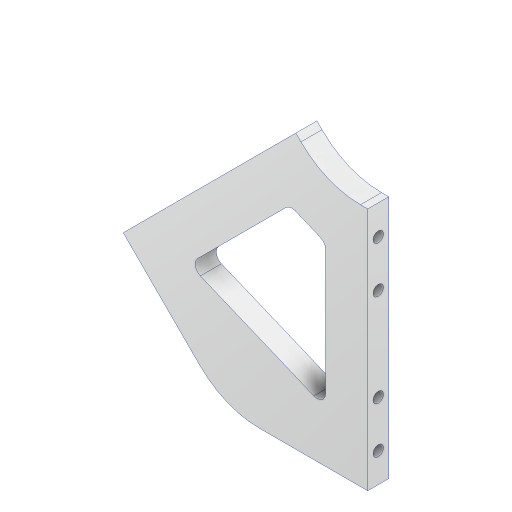
# Autodesk Inventor part: 조인트3_박스사이드_6T
Saved by Autodesk Inventor 2023.2 (Build 272271000, 271)
## iProperties
Created: 2022-01-24
Part Number: 조인트3_박스사이드_6T
Material: 알루미늄 6061
Document SubType Name: Modeling
Designer: BAEK
Density: 2.7 g/cm^3
Appearance: 알루미늄 - 평지
Mass: 29.5114 g
Surface Area: 59.5871 cm^2
Volume: 10.9301 cm^3
Author: BAEK
Autodesk Inventor part; units mm, degrees
ref_plane "YZ Plane" through (0, 0, 0) normal (1, 0, 0) x (0, 1, 0)
ref_plane "XZ Plane" through (0, 0, 0) normal (0, 1, 0) x (-1, 0, 0)
ref_plane "XY Plane" through (0, 0, 0) normal (0, 0, 1) x (1, 0, 0)
sketch "스케치1" plane through (0, 0, 0) normal (0, 0, 1) x (1, 0, 0)
  line L0 (0, 0) -> (0, 58)
  line L1 (0, 58) -> (-1.7157, 58)
  line L2 (-15.8579, 63.8579) -> (-17.0711, 65.0711)
  line L3 (-10, 58) -> (-8.2843, 58) construction
  line L4 (-17.0711, 65.0711) -> (-58.0833, 24.0589)
  line L5 (-58.0833, 24.0589) -> (-39.8823, 5.8579)
  line L6 (-25.7401, 0) -> (0, 0)
  arc A0 (-15.8579, 63.8579) -> (-1.7157, 58) centre (-1.7157, 78) ccw
  arc A1 (-39.8823, 5.8579) -> (-25.7401, 0) centre (-25.7401, 20) ccw
  point P0 (-34.0244, 0)
  dimension "d4" = 58
  dimension "d5" = 10
  dimension "d7" = 10
  dimension "d8" = 135
  dimension "d11" = 58
  dimension "d14" = 135
  dimension "d16" = 20
  dimension "d53" = 45
  constraints: 14 end point, 4 point on circle, 4 tangent, 2 centre point, 2 horizontal, 2 point on line, 1 equal length, 1 equal radius, 1 perpendicular, 1 vertical
  measures "d4" distance of L0.start L0.end
  measures "d5" distance of L0.end L3.start
  measures "d7" distance of L3.start L2.end
  measures "d8" angle of L3 L2
  measures "d11" distance of L2.end L4.end
  measures "d14" angle of L5 L6
  measures "d16" radius of A0
  measures "d53" angle of L0 L4
extrude "돌출1" add sketch "스케치1" along normal blind 5
sketch "스케치3" plane through (0, 0, 5) normal (0, 0, 1) x (1, 0, 0)
  line L0 (-19.4302, 48.5698) -> (-40.4104, 27.5896)
  line L1 (-17.0711, 65.0711) -> (-58.0833, 24.0589) projected
  line L2 (-58.0833, 24.0589) -> (-39.8823, 5.8579) projected
  line L3 (-15.8579, 63.8579) -> (-17.0711, 65.0711) projected
  line L4 (-10, 44.6636) -> (-10, 14.9932)
  line L5 (0, 58) -> (-1.7157, 58) projected
  line L6 (-25.7401, 0) -> (0, 0) projected
  line L7 (0, 0) -> (0, 58) projected
  line L8 (-39.7615, 24.3276) -> (-12.7654, 13.1455)
  line L9 (-11.2346, 46.5114) -> (-17.2506, 49.0033)
  arc A0 (-40.4104, 27.5896) -> (-39.7615, 24.3276) centre (-38.9962, 26.1754) ccw
  arc A1 (-12.7654, 13.1455) -> (-10, 14.9932) centre (-12, 14.9932) ccw
  arc A2 (-10, 44.6636) -> (-11.2346, 46.5114) centre (-12, 44.6636) ccw
  arc A3 (-17.2506, 49.0033) -> (-19.4302, 48.5698) centre (-18.016, 47.1556) ccw
  point P0 (-43.9411, 24.0589)
  point P1 (-36.8701, 16.9878)
  point P2 (-10, 10)
  point P3 (-20, 10)
  point P4 (-18.4853, 49.5147)
  point P5 (-42.5269, 25.4731)
  point P6 (-10, 46)
  point P7 (-10, 12)
  dimension "d17" = 10
  dimension "d20" = 10
  dimension "d23" = 10
  dimension "d24" = 10
  dimension "d52" = 2
  constraints: 10 point on line, 8 end point, 8 point on circle, 8 tangent, 4 centre point, 3 equal radius, 2 parallel
  measures "d17" distance between parallel lines of L1 L0
  measures "d20" distance of point (-43.941, 24.059) point (-36.87, 16.988)
  measures "d23" distance of point (-10, 10) point (-20, 10)
  measures "d24" distance between parallel lines of L7 L4
  measures "d52" radius of A0
extrude "돌출2" cut sketch "스케치3" against normal blind 6
sketch "스케치4" plane through (-58.0833, 24.0589, 0) normal (-0.7071, 0.7071, 0) x (-0.7071, -0.7071, 0)
  line L0 (-58, 0) -> (-58, 5) projected
  line L1 (-58, 2.5) -> (0, 2.5) construction
  line L2 (0, 0) -> (0, 5) projected
  circle A0 centre (-51, 2.5) radius 1.25
  circle A1 centre (-40, 2.5) radius 1.25
  circle A2 centre (-18, 2.5) radius 1.25
  circle A3 centre (-7, 2.5) radius 1.25
  point P0 (-24.0589, 0)
  dimension "d29" = 2.5
  dimension "d30" = 2.5
  dimension "d31" = 2.5
  dimension "d32" = 2.5
  dimension "d33" = 7
  dimension "d34" = 11
  dimension "d35" = 22
  dimension "d36" = 11
  constraints: 4 centre point, 4 point on line, 2 end point, 2 midpoint
  measures "d29" diameter of A0
  measures "d30" diameter of A1
  measures "d31" diameter of A2
  measures "d32" diameter of A3
  measures "d33" distance of L1.start A0.centre
  measures "d34" distance of A0.centre A1.centre
  measures "d35" distance of A1.centre A2.centre
  measures "d36" distance of A2.centre A3.centre
extrude "돌출3" cut sketch "스케치4" against normal blind 6
sketch "스케치5" plane through (0, 0, 0) normal (1, 0, 0) x (0, 0, -1)
  line L0 (0, 58) -> (-5, 58) projected
  line L1 (-2.5, 58) -> (-2.5, 17.6545) construction
  circle A0 centre (-2.5, 51) radius 1.25
  circle A1 centre (-2.5, 40) radius 1.25
  circle A2 centre (-2.5, 18) radius 1.25
  circle A3 centre (-2.5, 7) radius 1.25
  line L2 (0, 0) -> (-5, 0) projected
  dimension "d39" = 2.5
  dimension "d40" = 2.5
  dimension "d41" = 2.5
  dimension "d42" = 2.5
  dimension "d43" = 7
  dimension "d44" = 11
  dimension "d45" = 11
  dimension "d47" = 7
  constraints: 4 centre point, 4 point on line, 2 end point, 1 midpoint, 1 vertical
  measures "d39" diameter of A0
  measures "d40" diameter of A1
  measures "d41" diameter of A2
  measures "d42" diameter of A3
  measures "d43" distance from line of L0 A0.centre
  measures "d44" distance of A0.centre A1.centre
  measures "d45" distance of A3.centre A2.centre
  measures "d47" distance from line of L2 A3.centre
extrude "돌출4" cut sketch "스케치5" against normal blind 6
sketch "스케치6" plane through (0, 0, 0) normal (1, 0, 0) x (0, 0, -1)
  circle A0 centre (-2.5, 40) radius 1.25 projected
  circle A1 centre (-2.5, 18) radius 1.25 projected
  circle A2 centre (-2.5, 51) radius 1.25 projected
  circle A3 centre (-2.5, 7) radius 1.25 projected
  line L0 (0, 0) -> (0, 58) projected
  line L1 (0, 58) -> (-5, 58) projected
  line L2 (-5, 0) -> (-5, 58) projected
  line L3 (0, 0) -> (-5, 0) projected
